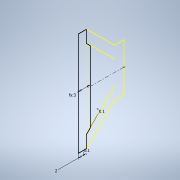
# Autodesk Inventor part: hopper lid
Saved by Autodesk Inventor 2022 (Build 260153000, 153)
## iProperties
Created: 2022-04-25
Part Number: hopper lid
Material: Generic
Document SubType Name: Modeling
Designer: efred
Density: 1 g/cm^3
Appearance: Default
Author: efred
Autodesk Inventor part; units mm, degrees
ref_plane "YZ Plane" through (0, 0, 0) normal (1, 0, 0) x (0, 1, 0)
ref_plane "Work Plane1" through (-12.4, -4.3, -12.7) normal (1, 0, 0) x (0, 1, 0)
sketch "Sketch1" plane through (0, 0, 0) normal (1, 0, 0) x (0, 1, 0)
  line L0 (16, -9.5) -> (16, -7.1) projected
  line L1 (16, -9.5) -> (4, -9.5) projected
  line L2 (4, -9.5) -> (4, -7.1) projected
  line L3 (-3, -0.1) -> (4, -7.1) projected
  line L4 (23, -0.1) -> (-3, -0.1) construction
  line L5 (16, -7.1) -> (23, -0.1) projected
  line L6 (13, -7.1) -> (20, -0.1) projected
  line L7 (0, -0.1) -> (7, -7.1) projected
  line L8 (0.0414, 0) -> (1.0414, -1)
  line L9 (0.0414, 0) -> (-3, 0)
  line L10 (-3, 0) -> (-3, 2)
  line L11 (-3, 2) -> (10, 2)
  line L12 (10, -9.5) -> (10, 0) construction
  line L13 (1.0414, -1) -> (10, -1)
  line L14 (19.9586, 0) -> (18.9586, -1)
  line L15 (19.9586, 0) -> (23, 0)
  line L16 (23, 0) -> (23, 2)
  line L17 (23, 2) -> (10, 2)
  line L18 (18.9586, -1) -> (10, -1)
  point P0 (0, 0)
  dimension "d0" = 0.1
  dimension "d1" = 0.1
  dimension "d2" = 2
  dimension "d3" = 3
  constraints: 22 end point, 4 symmetric about line, 3 perpendicular, 2 midpoint, 2 parallel, 2 vertical alignment, 1 coincident, 1 horizontal, 1 point on line
  measures "d0" distance between parallel lines of L7 L8
  measures "d1" distance between parallel lines of L4 L9
  measures "d2" distance between parallel lines of L11 L9
  measures "d3" distance from line of L11 L8.end
extrude "Extrusion1" add sketch "Sketch1" against normal up to surface (12.4 mm away)
sketch "Sketch2" plane through (-12.4, -3, 2) normal (-1, 0, 0) x (0, 0, 1)
  line L0 (-3, 21.9586) -> (-3, 4.0414) projected
  line L1 (-3, 4.0414) -> (-2, 3.0414) projected
  line L2 (-2, 3.0414) -> (-2, 0) projected
  line L3 (-2, 0) -> (0, 0) projected
  line L4 (0, 0) -> (0, 26) projected
  line L5 (0, 26) -> (-2, 26) projected
  line L6 (-2, 26) -> (-2, 22.9586) projected
  line L7 (-2, 22.9586) -> (-3, 21.9586) projected
  line L8 (0, 26) -> (0, 0) projected
  line L9 (-2, 0) -> (0, 0)
  line L10 (0, 0) -> (0, 26)
  line L11 (0, 26) -> (-2, 26)
  line L12 (-2, 26) -> (-2, 0)
  point P0 (-2, 3)
  point P1 (-2, 3.0414)
  constraints: 8 end point, 2 parallel, 1 horizontal, 1 perpendicular
ref_plane "Work Plane2" through (-14.9, -3, -9.5) normal (-1, 0, 0) x (0, 0, 1)
extrude "Extrusion2" add sketch "Sketch2" along normal up to surface (2.5 mm away) contours L6 L5 L4 L3 L2 L12
mirror "Mirror1" about plane through (0, 10, 0.5) normal (1, 0, 0) of "Extrusion2", "Extrusion1"
sketch "Sketch3" plane through (-14.9, -3, 2) normal (0, 0, 1) x (1, 0, 0)
  line L0 (0, 0) -> (29.8, 0) projected
  line L1 (29.8, 26) -> (29.8, 0) projected
  line L2 (0, 26) -> (29.8, 26) projected
  line L3 (0, 26) -> (0, 0) projected
  circle A0 centre (14.9, 13) radius 1.35
  point P0 (14.9, 3)
  point P1 (0, 13)
  point P2 (14.9, 26)
  dimension "d8" = 2.7
  constraints: 2 midpoint, 1 centre point, 1 horizontal alignment, 1 vertical alignment
  measures "d8" diameter of A0
extrude "Extrusion3" cut sketch "Sketch3" against normal through all contours A0
body "Solid1"
